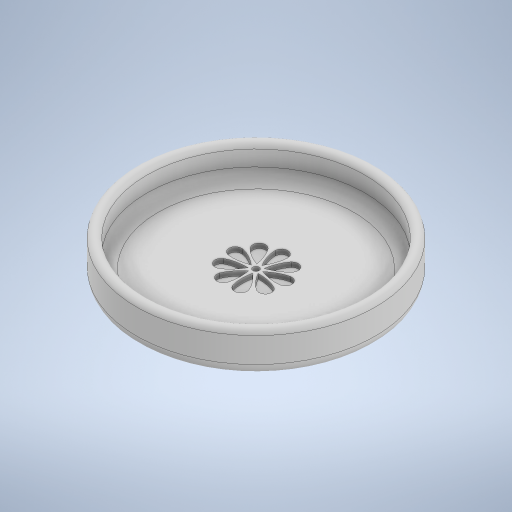
# Autodesk Inventor part: Plant Coaster V1
Saved by Autodesk Inventor 2024 (Build 280153000, 153)
## iProperties
Created: 2024-04-11
Part Number: Plant Coaster V1
Material: Generic
Document SubType Name: Modeling
Designer: haque
Density: 1 g/cm^3
Appearance: Default
Author: haque
Autodesk Inventor part; units mm, degrees
ref_plane "YZ Plane" through (0, 0, 0) normal (1, 0, 0) x (0, 1, 0)
ref_plane "XZ Plane" through (0, 0, 0) normal (0, 1, 0) x (-1, 0, 0)
ref_plane "XY Plane" through (0, 0, 0) normal (0, 0, 1) x (1, 0, 0)
sketch "Sketch1" plane through (0, 0, 0) normal (0, 1, 0) x (-1, 0, 0)
  circle A0 centre (0, 0) radius 37.5
  circle A1 centre (0, 0) radius 34.25
  dimension "d0" = 75
  dimension "d1" = 68.5
  constraints: 2 centre point, 2 coincident
  measures "d0" diameter of A0
  measures "d1" diameter of A1
extrude "Extrusion1" add sketch "Sketch1" along normal blind 13
extrude "Extrusion2" add sketch "Sketch1" along normal blind 3 contours A1
fillet "Fillet2" radius 3.5 2 edges at (34.25, 3, 0) (37.5, 0, 0)
fillet "Fillet3" radius 1.625 2 edges at (34.25, 13, 0) (37.5, 13, 0)
sketch "Sketch2" plane through (0, 3, 0) normal (0, 1, 0) x (1, 0, 0)
  circle A0 centre (0, 0) radius 10
  circle A1 centre (0, 0) radius 1
  line L0 (0, 0) -> (0, 10)
  circle A2 centre (0, 8) radius 2
  line L1 (2, 6) -> (-2, 6)
  line L2 (1, 3.5) -> (-1, 3.5)
  line L3 (0, 3.5) -> (0, -0.25)
  line L4 (0, 3.5) -> (0, 1.8333)
  line L5 (-2, 8) -> (-2, 6) construction
  line L6 (-2, 6) -> (-1, 3.5) construction
  line L7 (-1, 3.5) -> (0, 1.8333) construction
  spline S0 degree 3 poles (-2, 8) (-2, 6) (-1, 3.5) (0, 1.8333) knots 1 1 1 1 2 2 2 2
  line L8 (2, 8) -> (2, 6) construction
  line L9 (2, 6) -> (1, 3.5) construction
  line L10 (1, 3.5) -> (0, 1.8333) construction
  spline S1 degree 3 poles (2, 8) (2, 6) (1, 3.5) (0, 1.8333) knots 1 1 1 1 2 2 2 2
  dimension "d9" = 20
  dimension "d10" = 2
  dimension "d11" = 4
  constraints: 10 end point, 6 coincident, 3 point on line, 2 centre point, 2 point on circle, 2 tangent, 1 midpoint, 1 parallel, 1 perpendicular, 1 vertical, 1 vertical alignment, 8 other
  measures "d10" diameter of A1
  measures "d11" diameter of A2
extrude "Extrusion3" cut sketch "Sketch2" against normal blind 1.5 contours A2 L0 | L0 A2 | L1 S1 L2 L0 | L1 S0 A2 | A2 S1 L1 | L0 L2 S0 L1 | L2 S1 L0 | L0 S0 L2 | A1
pattern_circular "Circular Pattern1" count 9 over 360 about axis through (0, -10, 0) along (0, 1, 0) of "Extrusion3"
body "Solid1"
